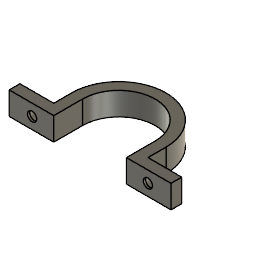
Saddle Clamp (Autodesk Fusion 360 design; units mm, degrees)
part number: 2026-04-02-17-03-18-147
Autodesk Fusion 360 part; units mm, degrees
note: some values were not read from the file. Set by a fixed rule: which sketch regions a step uses.
sketch "Sketch1" plane through (0, 0, 0) normal (0, 0, 1) x (1, 0, 0)
  line L0 (0, 0) -> (0, 25.1) construction
  line L1 (-28.1, 2.5) -> (-12.6, 2.5)
  line L2 (-12.6, 2.5) -> (-12.6, 12.6)
  line L3 (-16.3497, 12.6) -> (-28.1, 12.6)
  line L4 (-28.1, 12.6) -> (-28.1, 2.5)
  line L5 (28.1, 12.6) -> (28.1, 2.5)
  line L6 (16.3497, 12.6) -> (28.1, 12.6)
  line L7 (28.1, 2.5) -> (12.6, 2.5)
  line L8 (12.6, 2.5) -> (12.6, 12.6)
  arc A0 (16.3497, 12.6) -> (-16.3497, 12.6) centre (0, 12.5) ccw
  arc A1 (12.6, 12.5) -> (-12.6, 12.5) centre (0, 12.5) ccw
  line L9 (-28.1, 12.6) -> (-16.35, 12.6)
  line L10 (-16.35, 12.6) -> (-16.35, 6.25)
  line L11 (-16.35, 6.25) -> (-28.1, 6.25)
  line L12 (-28.1, 6.25) -> (-28.1, 12.6)
  line L13 (28.1, 12.6) -> (16.35, 12.6)
  line L14 (16.35, 6.25) -> (28.1, 6.25)
  line L15 (16.35, 12.6) -> (16.35, 6.25)
  point P0 (0, 12.5)
  point P1 (-12.6, 12.6)
  point P2 (-28.1, 2.5)
  point P3 (12.6, 12.6)
  point P4 (-28.1, 2.5)
  point P5 (-20.1, 6.15)
  point P6 (-16.35, 12.5)
  point P7 (20.1, 6.15)
  dimension "d1" = 25.2
  dimension "d2" = 32.7
  dimension "d3" = 11.75
  dimension "d4" = 6.35
  constraint coincident P0 A0.centre
  constraint coincident L0.start origin
  constraint coincident L0.end A1
  constraint vertical L0
  constraint symmetric P1 L0 L8.end
  constraint horizontal L1
  constraint vertical L2
  constraint horizontal L3
  constraint vertical L4
  constraint coincident P1 L2.end
  constraint coincident P2 L1.start
  constraint symmetric L0 P4 L5.end
  constraint symmetric L0 L1.end L7.end
  constraint symmetric L0 P1 P3
  constraint symmetric L0 L3.end L5.start
  constraint concentric A0 A1
  constraint coincident L2 A1.end
  constraint coincident L8 A1.start
  constraint horizontal L9
  constraint vertical L10
  constraint horizontal L11
  constraint vertical L12
  constraint symmetric L0 L9.end L13.end
  constraint symmetric L0 L10.end L14.start
  constraint symmetric L0 L11.end L14.end
  constraint symmetric L0 P5 P7
  measures "d1" diameter of A1
  measures "d2" diameter of A0
  measures "d3" distance of L3.end L9.end
  measures "d4" distance of L3.end L11.end
extrude "Extrude1" add sketch "Sketch1" along normal blind 8 contours L1 L2 L4 L5 L7 L8 A0 A1 L10 L11 L14 L15
sketch "Sketch2" plane through (0, 6.25, 0) normal (0, 1, 0) x (-1, 0, 0)
  line L0 (16.35, 0) -> (28.1, 0)
  line L1 (28.1, 0) -> (28.1, 8)
  line L2 (28.1, 8) -> (16.35, 8)
  line L3 (16.35, 8) -> (16.35, 0)
  line L4 (0, 8) -> (0, 0) construction
  point P0 (20.1, 4)
  point P1 (-20.1, 4)
  constraint coincident L4.end origin
  constraint vertical L4
  constraint symmetric P0 L4 P1
hole "Hole1" at (-20.1, 6.25, 4) at (20.1, 6.25, 4) direction (0, -1, 0) diameter 3.2 end through all counterbore diameter 6 counterbore depth 3
